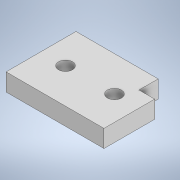
# Autodesk Inventor part: gantryBeltCnctr
Saved by Autodesk Inventor 2022 (Build 260153000, 153)
## iProperties
Created: 2022-04-01
Part Number: gantryBeltCnctr
Material: Generic
Document SubType Name: Modeling
Designer: Phabryan
Density: 1 g/cm^3
Appearance: Default
Author: Phabryan
Autodesk Inventor part; units mm, degrees
ref_plane "YZ Plane" through (0, 0, 0) normal (1, 0, 0) x (0, 1, 0)
ref_plane "XZ Plane" through (0, 0, 0) normal (0, 1, 0) x (-1, 0, 0)
ref_plane "XY Plane" through (0, 0, 0) normal (0, 0, 1) x (1, 0, 0)
sketch "Sketch1" plane through (0, 0, 0) normal (0, 1, 0) x (-1, 0, 0)
  point P0 (0, 0)
sketch "Sketch2" plane through (0, 0, 0) normal (0, 1, 0) x (-1, 0, 0)
  line L0 (14, 10) -> (-14, 10)
  line L1 (-14, 10) -> (-14, -10)
  line L2 (-14, -10) -> (14, -10)
  line L3 (14, -10) -> (14, 10)
  point P0 (0, 0)
  dimension "d0" = 28
  dimension "d1" = 20
  constraints: 8 end point, 2 parallel, 1 horizontal, 1 perpendicular
  measures "d0" distance of L2.end L1.end
  measures "d1" distance of L1.end L0.end
extrude "Extrusion1" add sketch "Sketch2" along normal blind 5
sketch "Sketch3" plane through (0, 5, 0) normal (0, 1, 0) x (1, 0, 0)
  circle A0 centre (7, 0) radius 2
  circle A1 centre (-7, 0) radius 2
  point P0 (0, 0)
  dimension "d4" = 4
  dimension "d5" = 4
  constraints: 2 centre point
  measures "d4" diameter of A0
  measures "d5" diameter of A1
extrude "Extrusion2" cut sketch "Sketch3" against normal blind 6
sketch "Sketch4" plane through (0, 5, 0) normal (0, 1, 0) x (1, 0, 0)
  line L0 (9.5, 4.5) -> (16.3647, 4.5)
  line L1 (16.3647, 4.5) -> (16.3647, 12.8099)
  line L2 (16.3647, 12.8099) -> (9.5, 12.8099)
  line L3 (9.5, 12.8099) -> (9.5, 4.5)
  point P0 (0, 0)
  constraints: 8 end point, 2 parallel, 1 horizontal, 1 perpendicular
extrude "Extrusion3" cut sketch "Sketch4" against normal blind 6
body "Solid1"
